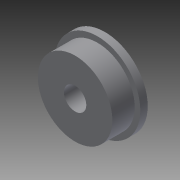
# Autodesk Inventor part: bearing flanged 10x3x4mm
Saved by Autodesk Inventor 2013 SP2 (Build 170200200, 200)
## iProperties
Created: 2017-05-18
Part Number: bearing flanged 10x3x4mm
Material: Generic
Document SubType Name: Modeling
Designer: Herman de Vries
Density: 1 g/cm^3
Author: Herman de Vries
Autodesk Inventor part; units mm, degrees
ref_plane "YZ Plane" through (0, 0, 0) normal (1, 0, 0) x (0, 1, 0)
ref_plane "XZ Plane" through (0, 0, 0) normal (0, 1, 0) x (-1, 0, 0)
ref_plane "XY Plane" through (0, 0, 0) normal (0, 0, 1) x (1, 0, 0)
sketch "Sketch1" plane through (0, 0, 0) normal (0, 0, 1) x (1, 0, 0)
  line L0 (1.5, 0) -> (5, 0)
  line L1 (5, 0) -> (5, 4)
  line L2 (5, 4) -> (1.5, 4)
  line L3 (1.5, 4) -> (1.5, 0)
  line L4 (5, 4) -> (5.75, 4)
  line L5 (5.75, 4) -> (5.75, 3)
  line L6 (5.75, 3) -> (5, 3)
  line L7 (5, 3) -> (5, 4)
  line L8 (0, 0) -> (0, 6.6481) construction
  dimension "d0" = 1.5
  dimension "d1" = 5
  dimension "d2" = 0.75
  dimension "d3" = 4
  dimension "d4" = 1
  constraints: 18 end point, 5 parallel, 2 horizontal, 2 perpendicular, 1 horizontal alignment
  measures "d0" distance from line of L3 L8.start
  measures "d1" distance from line of L1 L8.start
  measures "d2" distance between parallel lines of L5 L1
  measures "d3" distance between parallel lines of L2 L0
  measures "d4" distance of L4.end L5.end
revolve "Revolution1" add sketch "Sketch1" angle 360 about axis through (0, 0, 0) along (0, 1, 0)
body "Solid1"
